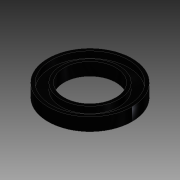
# Autodesk Inventor part: Cap
Saved by Autodesk Inventor 2014 SP1 (Build 180222100, 222)
## iProperties
Created: 2017-07-23
Part Number: Cap
Material: Типовые
Document SubType Name: Modeling
Designer: Stepan
Density: 1 g/cm^3
Appearance: С гладкой текстурой — черный
Author: Stepan
Autodesk Inventor part; units mm, degrees
ref_plane "YZ Plane" through (0, 0, 0) normal (1, 0, 0) x (0, 1, 0)
ref_plane "XZ Plane" through (0, 0, 0) normal (0, 1, 0) x (-1, 0, 0)
ref_plane "XY Plane" through (0, 0, 0) normal (0, 0, 1) x (1, 0, 0)
sketch "Эскиз1" plane through (0, 0, 0) normal (0, 0, 1) x (1, 0, 0)
  circle A0 centre (0, 0) radius 4 projected
  circle A1 centre (0, 0) radius 6.5 projected
extrude "Выдавливание1" add sketch "Эскиз1" along normal blind 1
sketch "Эскиз2" plane through (0, 0, 1) normal (0, 0, 1) x (1, 0, 0)
  circle A0 centre (0, 0) radius 4 projected
  circle A1 centre (0, 0) radius 6.5 projected
  circle A2 centre (0, 0) radius 6
  circle A3 centre (0, 0) radius 4.5
  dimension "d2" = 12
  dimension "d3" = 9
  constraints: 2 centre point, 2 coincident
  measures "d2" diameter of A2
  measures "d3" diameter of A3
extrude "Выдавливание2" add sketch "Эскиз2" along normal blind 0.7
